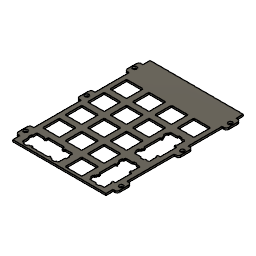
Plate (Autodesk Fusion 360 design; units mm, degrees)
part number: 2026-08-19-10-44-33-634
Autodesk Fusion 360 part; units mm, degrees
sketch "plate-2026-08-19T09_43_30.871Z" plane through (0, 0, 0) normal (0, 0, 1) x (1, 0, 0)
  line L0 (3.025, -2.525) -> (16.025, -2.525)
  line L1 (3.025, -16.525) -> (16.025, -16.525)
  line L2 (2.525, -3.025) -> (2.525, -16.025)
  line L3 (16.525, -3.025) -> (16.525, -16.025)
  arc A0 (3.025, -2.525) -> (2.525, -3.025) centre (3.025, -3.025) ccw
  arc A1 (16.525, -3.025) -> (16.025, -2.525) centre (16.025, -3.025) ccw
  arc A2 (2.525, -16.025) -> (3.025, -16.525) centre (3.025, -16.025) ccw
  arc A3 (16.025, -16.525) -> (16.525, -16.025) centre (16.025, -16.025) ccw
  line L4 (22.075, -2.525) -> (35.075, -2.525)
  line L5 (22.075, -16.525) -> (35.075, -16.525)
  line L6 (21.575, -3.025) -> (21.575, -16.025)
  line L7 (35.575, -3.025) -> (35.575, -16.025)
  arc A4 (22.075, -2.525) -> (21.575, -3.025) centre (22.075, -3.025) ccw
  arc A5 (35.575, -3.025) -> (35.075, -2.525) centre (35.075, -3.025) ccw
  arc A6 (21.575, -16.025) -> (22.075, -16.525) centre (22.075, -16.025) ccw
  arc A7 (35.075, -16.525) -> (35.575, -16.025) centre (35.075, -16.025) ccw
  line L8 (41.125, -2.525) -> (54.125, -2.525)
  line L9 (41.125, -16.525) -> (54.125, -16.525)
  line L10 (40.625, -3.025) -> (40.625, -16.025)
  line L11 (54.625, -3.025) -> (54.625, -16.025)
  arc A8 (41.125, -2.525) -> (40.625, -3.025) centre (41.125, -3.025) ccw
  arc A9 (54.625, -3.025) -> (54.125, -2.525) centre (54.125, -3.025) ccw
  arc A10 (40.625, -16.025) -> (41.125, -16.525) centre (41.125, -16.025) ccw
  arc A11 (54.125, -16.525) -> (54.625, -16.025) centre (54.125, -16.025) ccw
  line L12 (60.175, -2.525) -> (73.175, -2.525)
  line L13 (60.175, -16.525) -> (73.175, -16.525)
  line L14 (59.675, -3.025) -> (59.675, -16.025)
  line L15 (73.675, -3.025) -> (73.675, -16.025)
  arc A12 (60.175, -2.525) -> (59.675, -3.025) centre (60.175, -3.025) ccw
  arc A13 (73.675, -3.025) -> (73.175, -2.525) centre (73.175, -3.025) ccw
  arc A14 (59.675, -16.025) -> (60.175, -16.525) centre (60.175, -16.025) ccw
  arc A15 (73.175, -16.525) -> (73.675, -16.025) centre (73.175, -16.025) ccw
  line L16 (3.025, -21.575) -> (16.025, -21.575)
  line L17 (3.025, -35.575) -> (16.025, -35.575)
  line L18 (2.525, -22.075) -> (2.525, -35.075)
  line L19 (16.525, -22.075) -> (16.525, -35.075)
  arc A16 (3.025, -21.575) -> (2.525, -22.075) centre (3.025, -22.075) ccw
  arc A17 (16.525, -22.075) -> (16.025, -21.575) centre (16.025, -22.075) ccw
  arc A18 (2.525, -35.075) -> (3.025, -35.575) centre (3.025, -35.075) ccw
  arc A19 (16.025, -35.575) -> (16.525, -35.075) centre (16.025, -35.075) ccw
  line L20 (22.075, -21.575) -> (35.075, -21.575)
  line L21 (22.075, -35.575) -> (35.075, -35.575)
  line L22 (21.575, -22.075) -> (21.575, -35.075)
  line L23 (35.575, -22.075) -> (35.575, -35.075)
  arc A20 (22.075, -21.575) -> (21.575, -22.075) centre (22.075, -22.075) ccw
  arc A21 (35.575, -22.075) -> (35.075, -21.575) centre (35.075, -22.075) ccw
  arc A22 (21.575, -35.075) -> (22.075, -35.575) centre (22.075, -35.075) ccw
  arc A23 (35.075, -35.575) -> (35.575, -35.075) centre (35.075, -35.075) ccw
  line L24 (41.125, -21.575) -> (54.125, -21.575)
  line L25 (41.125, -35.575) -> (54.125, -35.575)
  line L26 (40.625, -22.075) -> (40.625, -35.075)
  line L27 (54.625, -22.075) -> (54.625, -35.075)
  arc A24 (41.125, -21.575) -> (40.625, -22.075) centre (41.125, -22.075) ccw
  arc A25 (54.625, -22.075) -> (54.125, -21.575) centre (54.125, -22.075) ccw
  arc A26 (40.625, -35.075) -> (41.125, -35.575) centre (41.125, -35.075) ccw
  arc A27 (54.125, -35.575) -> (54.625, -35.075) centre (54.125, -35.075) ccw
  line L28 (73.675, -31.6) -> (73.675, -44.6)
  line L29 (59.675, -31.6) -> (59.675, -44.6)
  line L30 (73.175, -31.1) -> (60.175, -31.1)
  line L31 (73.175, -45.1) -> (60.175, -45.1)
  arc A28 (73.675, -31.6) -> (73.175, -31.1) centre (73.175, -31.6) ccw
  arc A29 (73.175, -45.1) -> (73.675, -44.6) centre (73.175, -44.6) ccw
  arc A30 (60.175, -31.1) -> (59.675, -31.6) centre (60.175, -31.6) ccw
  arc A31 (59.675, -44.6) -> (60.175, -45.1) centre (60.175, -44.6) ccw
  line L32 (72.3646, -23.3346) -> (72.3646, -28.9894)
  line L33 (71.8646, -29.4894) -> (71.5518, -29.4894)
  line L34 (71.5518, -29.4894) -> (71.5518, -38.1)
  line L35 (60.8584, -38.1) -> (60.8584, -29.9894)
  line L36 (60.3584, -29.4894) -> (60.071, -29.4894)
  line L37 (60.071, -29.4894) -> (60.071, -28.186)
  line L38 (59.571, -27.686) -> (59.4026, -27.686)
  line L39 (58.9026, -27.186) -> (58.9026, -25.138)
  line L40 (59.4026, -24.638) -> (59.571, -24.638)
  line L41 (60.071, -24.138) -> (60.071, -23.3346)
  line L42 (60.571, -22.8346) -> (65.667, -22.8346)
  line L43 (66.167, -22.3346) -> (66.167, -21.971)
  line L44 (66.167, -21.971) -> (68.461, -21.971)
  line L45 (68.961, -22.471) -> (68.961, -22.8346)
  line L46 (68.961, -22.8346) -> (71.8646, -22.8346)
  arc A32 (71.8646, -29.4894) -> (72.3646, -28.9894) centre (71.8646, -28.9894) ccw
  arc A33 (60.8584, -29.9894) -> (60.3584, -29.4894) centre (60.3584, -29.9894) ccw
  arc A34 (60.071, -28.186) -> (59.571, -27.686) centre (59.571, -28.186) ccw
  arc A35 (58.9026, -27.186) -> (59.4026, -27.686) centre (59.4026, -27.186) ccw
  arc A36 (59.4026, -24.638) -> (58.9026, -25.138) centre (59.4026, -25.138) ccw
  arc A37 (59.571, -24.638) -> (60.071, -24.138) centre (59.571, -24.138) ccw
  arc A38 (60.571, -22.8346) -> (60.071, -23.3346) centre (60.571, -23.3346) ccw
  arc A39 (65.667, -22.8346) -> (66.167, -22.3346) centre (65.667, -22.3346) ccw
  arc A40 (68.961, -22.471) -> (68.461, -21.971) centre (68.461, -22.471) ccw
  arc A41 (72.3646, -23.3346) -> (71.8646, -22.8346) centre (71.8646, -23.3346) ccw
  line L47 (72.3646, -52.8654) -> (72.3646, -47.2106)
  line L48 (71.8646, -46.7106) -> (71.5518, -46.7106)
  line L49 (71.5518, -46.7106) -> (71.5518, -38.1)
  line L50 (60.8584, -38.1) -> (60.8584, -46.2106)
  line L51 (60.3584, -46.7106) -> (60.071, -46.7106)
  line L52 (60.071, -46.7106) -> (60.071, -48.014)
  line L53 (59.571, -48.514) -> (59.4026, -48.514)
  line L54 (58.9026, -49.014) -> (58.9026, -51.062)
  line L55 (59.4026, -51.562) -> (59.571, -51.562)
  line L56 (60.071, -52.062) -> (60.071, -52.8654)
  line L57 (60.571, -53.3654) -> (65.667, -53.3654)
  line L58 (66.167, -53.8654) -> (66.167, -54.229)
  line L59 (66.167, -54.229) -> (68.461, -54.229)
  line L60 (68.961, -53.729) -> (68.961, -53.3654)
  line L61 (68.961, -53.3654) -> (71.8646, -53.3654)
  arc A42 (72.3646, -47.2106) -> (71.8646, -46.7106) centre (71.8646, -47.2106) ccw
  arc A43 (60.3584, -46.7106) -> (60.8584, -46.2106) centre (60.3584, -46.2106) ccw
  arc A44 (59.571, -48.514) -> (60.071, -48.014) centre (59.571, -48.014) ccw
  arc A45 (59.4026, -48.514) -> (58.9026, -49.014) centre (59.4026, -49.014) ccw
  arc A46 (58.9026, -51.062) -> (59.4026, -51.562) centre (59.4026, -51.062) ccw
  arc A47 (60.071, -52.062) -> (59.571, -51.562) centre (59.571, -52.062) ccw
  arc A48 (60.071, -52.8654) -> (60.571, -53.3654) centre (60.571, -52.8654) ccw
  arc A49 (66.167, -53.8654) -> (65.667, -53.3654) centre (65.667, -53.8654) ccw
  arc A50 (68.461, -54.229) -> (68.961, -53.729) centre (68.461, -53.729) ccw
  arc A51 (71.8646, -53.3654) -> (72.3646, -52.8654) centre (71.8646, -52.8654) ccw
  line L62 (3.025, -40.625) -> (16.025, -40.625)
  line L63 (3.025, -54.625) -> (16.025, -54.625)
  line L64 (2.525, -41.125) -> (2.525, -54.125)
  line L65 (16.525, -41.125) -> (16.525, -54.125)
  arc A52 (3.025, -40.625) -> (2.525, -41.125) centre (3.025, -41.125) ccw
  arc A53 (16.525, -41.125) -> (16.025, -40.625) centre (16.025, -41.125) ccw
  arc A54 (2.525, -54.125) -> (3.025, -54.625) centre (3.025, -54.125) ccw
  arc A55 (16.025, -54.625) -> (16.525, -54.125) centre (16.025, -54.125) ccw
  line L66 (22.075, -40.625) -> (35.075, -40.625)
  line L67 (22.075, -54.625) -> (35.075, -54.625)
  line L68 (21.575, -41.125) -> (21.575, -54.125)
  line L69 (35.575, -41.125) -> (35.575, -54.125)
  arc A56 (22.075, -40.625) -> (21.575, -41.125) centre (22.075, -41.125) ccw
  arc A57 (35.575, -41.125) -> (35.075, -40.625) centre (35.075, -41.125) ccw
  arc A58 (21.575, -54.125) -> (22.075, -54.625) centre (22.075, -54.125) ccw
  arc A59 (35.075, -54.625) -> (35.575, -54.125) centre (35.075, -54.125) ccw
  line L70 (41.125, -40.625) -> (54.125, -40.625)
  line L71 (41.125, -54.625) -> (54.125, -54.625)
  line L72 (40.625, -41.125) -> (40.625, -54.125)
  line L73 (54.625, -41.125) -> (54.625, -54.125)
  arc A60 (41.125, -40.625) -> (40.625, -41.125) centre (41.125, -41.125) ccw
  arc A61 (54.625, -41.125) -> (54.125, -40.625) centre (54.125, -41.125) ccw
  arc A62 (40.625, -54.125) -> (41.125, -54.625) centre (41.125, -54.125) ccw
  arc A63 (54.125, -54.625) -> (54.625, -54.125) centre (54.125, -54.125) ccw
  line L74 (3.025, -59.675) -> (16.025, -59.675)
  line L75 (3.025, -73.675) -> (16.025, -73.675)
  line L76 (2.525, -60.175) -> (2.525, -73.175)
  line L77 (16.525, -60.175) -> (16.525, -73.175)
  arc A64 (3.025, -59.675) -> (2.525, -60.175) centre (3.025, -60.175) ccw
  arc A65 (16.525, -60.175) -> (16.025, -59.675) centre (16.025, -60.175) ccw
  arc A66 (2.525, -73.175) -> (3.025, -73.675) centre (3.025, -73.175) ccw
  arc A67 (16.025, -73.675) -> (16.525, -73.175) centre (16.025, -73.175) ccw
  line L78 (22.075, -59.675) -> (35.075, -59.675)
  line L79 (22.075, -73.675) -> (35.075, -73.675)
  line L80 (21.575, -60.175) -> (21.575, -73.175)
  line L81 (35.575, -60.175) -> (35.575, -73.175)
  arc A68 (22.075, -59.675) -> (21.575, -60.175) centre (22.075, -60.175) ccw
  arc A69 (35.575, -60.175) -> (35.075, -59.675) centre (35.075, -60.175) ccw
  arc A70 (21.575, -73.175) -> (22.075, -73.675) centre (22.075, -73.175) ccw
  arc A71 (35.075, -73.675) -> (35.575, -73.175) centre (35.075, -73.175) ccw
  line L82 (41.125, -59.675) -> (54.125, -59.675)
  line L83 (41.125, -73.675) -> (54.125, -73.675)
  line L84 (40.625, -60.175) -> (40.625, -73.175)
  line L85 (54.625, -60.175) -> (54.625, -73.175)
  arc A72 (41.125, -59.675) -> (40.625, -60.175) centre (41.125, -60.175) ccw
  arc A73 (54.625, -60.175) -> (54.125, -59.675) centre (54.125, -60.175) ccw
  arc A74 (40.625, -73.175) -> (41.125, -73.675) centre (41.125, -73.175) ccw
  arc A75 (54.125, -73.675) -> (54.625, -73.175) centre (54.125, -73.175) ccw
  line L86 (73.675, -69.7) -> (73.675, -82.7)
  line L87 (59.675, -69.7) -> (59.675, -82.7)
  line L88 (73.175, -69.2) -> (60.175, -69.2)
  line L89 (73.175, -83.2) -> (60.175, -83.2)
  arc A76 (73.675, -69.7) -> (73.175, -69.2) centre (73.175, -69.7) ccw
  arc A77 (73.175, -83.2) -> (73.675, -82.7) centre (73.175, -82.7) ccw
  arc A78 (60.175, -69.2) -> (59.675, -69.7) centre (60.175, -69.7) ccw
  arc A79 (59.675, -82.7) -> (60.175, -83.2) centre (60.175, -82.7) ccw
  line L90 (72.3646, -61.4346) -> (72.3646, -67.0894)
  line L91 (71.8646, -67.5894) -> (71.5518, -67.5894)
  line L92 (71.5518, -67.5894) -> (71.5518, -76.2)
  line L93 (60.8584, -76.2) -> (60.8584, -68.0894)
  line L94 (60.3584, -67.5894) -> (60.071, -67.5894)
  line L95 (60.071, -67.5894) -> (60.071, -66.286)
  line L96 (59.571, -65.786) -> (59.4026, -65.786)
  line L97 (58.9026, -65.286) -> (58.9026, -63.238)
  line L98 (59.4026, -62.738) -> (59.571, -62.738)
  line L99 (60.071, -62.238) -> (60.071, -61.4346)
  line L100 (60.571, -60.9346) -> (65.667, -60.9346)
  line L101 (66.167, -60.4346) -> (66.167, -60.071)
  line L102 (66.167, -60.071) -> (68.461, -60.071)
  line L103 (68.961, -60.571) -> (68.961, -60.9346)
  line L104 (68.961, -60.9346) -> (71.8646, -60.9346)
  arc A80 (71.8646, -67.5894) -> (72.3646, -67.0894) centre (71.8646, -67.0894) ccw
  arc A81 (60.8584, -68.0894) -> (60.3584, -67.5894) centre (60.3584, -68.0894) ccw
  arc A82 (60.071, -66.286) -> (59.571, -65.786) centre (59.571, -66.286) ccw
  arc A83 (58.9026, -65.286) -> (59.4026, -65.786) centre (59.4026, -65.286) ccw
  arc A84 (59.4026, -62.738) -> (58.9026, -63.238) centre (59.4026, -63.238) ccw
  arc A85 (59.571, -62.738) -> (60.071, -62.238) centre (59.571, -62.238) ccw
  arc A86 (60.571, -60.9346) -> (60.071, -61.4346) centre (60.571, -61.4346) ccw
  arc A87 (65.667, -60.9346) -> (66.167, -60.4346) centre (65.667, -60.4346) ccw
  arc A88 (68.961, -60.571) -> (68.461, -60.071) centre (68.461, -60.571) ccw
  arc A89 (72.3646, -61.4346) -> (71.8646, -60.9346) centre (71.8646, -61.4346) ccw
  line L105 (72.3646, -90.9654) -> (72.3646, -85.3106)
  line L106 (71.8646, -84.8106) -> (71.5518, -84.8106)
  line L107 (71.5518, -84.8106) -> (71.5518, -76.2)
  line L108 (60.8584, -76.2) -> (60.8584, -84.3106)
  line L109 (60.3584, -84.8106) -> (60.071, -84.8106)
  line L110 (60.071, -84.8106) -> (60.071, -86.114)
  line L111 (59.571, -86.614) -> (59.4026, -86.614)
  line L112 (58.9026, -87.114) -> (58.9026, -89.162)
  line L113 (59.4026, -89.662) -> (59.571, -89.662)
  line L114 (60.071, -90.162) -> (60.071, -90.9654)
  line L115 (60.571, -91.4654) -> (65.667, -91.4654)
  line L116 (66.167, -91.9654) -> (66.167, -92.329)
  line L117 (66.167, -92.329) -> (68.461, -92.329)
  line L118 (68.961, -91.829) -> (68.961, -91.4654)
  line L119 (68.961, -91.4654) -> (71.8646, -91.4654)
  arc A90 (72.3646, -85.3106) -> (71.8646, -84.8106) centre (71.8646, -85.3106) ccw
  arc A91 (60.3584, -84.8106) -> (60.8584, -84.3106) centre (60.3584, -84.3106) ccw
  arc A92 (59.571, -86.614) -> (60.071, -86.114) centre (59.571, -86.114) ccw
  arc A93 (59.4026, -86.614) -> (58.9026, -87.114) centre (59.4026, -87.114) ccw
  arc A94 (58.9026, -89.162) -> (59.4026, -89.662) centre (59.4026, -89.162) ccw
  arc A95 (60.071, -90.162) -> (59.571, -89.662) centre (59.571, -90.162) ccw
  arc A96 (60.071, -90.9654) -> (60.571, -91.4654) centre (60.571, -90.9654) ccw
  arc A97 (66.167, -91.9654) -> (65.667, -91.4654) centre (65.667, -91.9654) ccw
  arc A98 (68.461, -92.329) -> (68.961, -91.829) centre (68.461, -91.829) ccw
  arc A99 (71.8646, -91.4654) -> (72.3646, -90.9654) centre (71.8646, -90.9654) ccw
  line L120 (12.55, -78.725) -> (25.55, -78.725)
  line L121 (12.55, -92.725) -> (25.55, -92.725)
  line L122 (12.05, -79.225) -> (12.05, -92.225)
  line L123 (26.05, -79.225) -> (26.05, -92.225)
  arc A100 (12.55, -78.725) -> (12.05, -79.225) centre (12.55, -79.225) ccw
  arc A101 (26.05, -79.225) -> (25.55, -78.725) centre (25.55, -79.225) ccw
  arc A102 (12.05, -92.225) -> (12.55, -92.725) centre (12.55, -92.225) ccw
  arc A103 (25.55, -92.725) -> (26.05, -92.225) centre (25.55, -92.225) ccw
  line L124 (4.2846, -80.0354) -> (9.9394, -80.0354)
  line L125 (10.4394, -80.5354) -> (10.4394, -80.8482)
  line L126 (10.4394, -80.8482) -> (19.05, -80.8482)
  line L127 (19.05, -91.5416) -> (10.9394, -91.5416)
  line L128 (10.4394, -92.0416) -> (10.4394, -92.329)
  line L129 (10.4394, -92.329) -> (9.136, -92.329)
  line L130 (8.636, -92.829) -> (8.636, -92.9974)
  line L131 (8.136, -93.4974) -> (6.088, -93.4974)
  line L132 (5.588, -92.9974) -> (5.588, -92.829)
  line L133 (5.088, -92.329) -> (4.2846, -92.329)
  line L134 (3.7846, -91.829) -> (3.7846, -86.733)
  line L135 (3.2846, -86.233) -> (2.921, -86.233)
  line L136 (2.921, -86.233) -> (2.921, -83.939)
  line L137 (3.421, -83.439) -> (3.7846, -83.439)
  line L138 (3.7846, -83.439) -> (3.7846, -80.5354)
  arc A104 (10.4394, -80.5354) -> (9.9394, -80.0354) centre (9.9394, -80.5354) ccw
  arc A105 (10.9394, -91.5416) -> (10.4394, -92.0416) centre (10.9394, -92.0416) ccw
  arc A106 (9.136, -92.329) -> (8.636, -92.829) centre (9.136, -92.829) ccw
  arc A107 (8.136, -93.4974) -> (8.636, -92.9974) centre (8.136, -92.9974) ccw
  arc A108 (5.588, -92.9974) -> (6.088, -93.4974) centre (6.088, -92.9974) ccw
  arc A109 (5.588, -92.829) -> (5.088, -92.329) centre (5.088, -92.829) ccw
  arc A110 (3.7846, -91.829) -> (4.2846, -92.329) centre (4.2846, -91.829) ccw
  arc A111 (3.7846, -86.733) -> (3.2846, -86.233) centre (3.2846, -86.733) ccw
  arc A112 (3.421, -83.439) -> (2.921, -83.939) centre (3.421, -83.939) ccw
  arc A113 (4.2846, -80.0354) -> (3.7846, -80.5354) centre (4.2846, -80.5354) ccw
  line L139 (33.8154, -80.0354) -> (28.1606, -80.0354)
  line L140 (27.6606, -80.5354) -> (27.6606, -80.8482)
  line L141 (27.6606, -80.8482) -> (19.05, -80.8482)
  line L142 (19.05, -91.5416) -> (27.1606, -91.5416)
  line L143 (27.6606, -92.0416) -> (27.6606, -92.329)
  line L144 (27.6606, -92.329) -> (28.964, -92.329)
  line L145 (29.464, -92.829) -> (29.464, -92.9974)
  line L146 (29.964, -93.4974) -> (32.012, -93.4974)
  line L147 (32.512, -92.9974) -> (32.512, -92.829)
  line L148 (33.012, -92.329) -> (33.8154, -92.329)
  line L149 (34.3154, -91.829) -> (34.3154, -86.733)
  line L150 (34.8154, -86.233) -> (35.179, -86.233)
  line L151 (35.179, -86.233) -> (35.179, -83.939)
  line L152 (34.679, -83.439) -> (34.3154, -83.439)
  line L153 (34.3154, -83.439) -> (34.3154, -80.5354)
  arc A114 (28.1606, -80.0354) -> (27.6606, -80.5354) centre (28.1606, -80.5354) ccw
  arc A115 (27.6606, -92.0416) -> (27.1606, -91.5416) centre (27.1606, -92.0416) ccw
  arc A116 (29.464, -92.829) -> (28.964, -92.329) centre (28.964, -92.829) ccw
  arc A117 (29.464, -92.9974) -> (29.964, -93.4974) centre (29.964, -92.9974) ccw
  arc A118 (32.012, -93.4974) -> (32.512, -92.9974) centre (32.012, -92.9974) ccw
  arc A119 (33.012, -92.329) -> (32.512, -92.829) centre (33.012, -92.829) ccw
  arc A120 (33.8154, -92.329) -> (34.3154, -91.829) centre (33.8154, -91.829) ccw
  arc A121 (34.8154, -86.233) -> (34.3154, -86.733) centre (34.8154, -86.733) ccw
  arc A122 (35.179, -83.939) -> (34.679, -83.439) centre (34.679, -83.939) ccw
  arc A123 (34.3154, -80.5354) -> (33.8154, -80.0354) centre (33.8154, -80.5354) ccw
  line L154 (41.125, -78.725) -> (54.125, -78.725)
  line L155 (41.125, -92.725) -> (54.125, -92.725)
  line L156 (40.625, -79.225) -> (40.625, -92.225)
  line L157 (54.625, -79.225) -> (54.625, -92.225)
  arc A124 (41.125, -78.725) -> (40.625, -79.225) centre (41.125, -79.225) ccw
  arc A125 (54.625, -79.225) -> (54.125, -78.725) centre (54.125, -79.225) ccw
  arc A126 (40.625, -92.225) -> (41.125, -92.725) centre (41.125, -92.225) ccw
  arc A127 (54.125, -92.725) -> (54.625, -92.225) centre (54.125, -92.225) ccw
  line L158 (0, -95.25) -> (76.2, -95.25)
  line L159 (0, 0) -> (76.2, 0)
  line L160 (0, -95.25) -> (0, 0)
  line L161 (76.2, -95.25) -> (76.2, 0)
sketch "Sketch2" plane through (0, 0, 0) normal (0, 0, 1) x (1, 0, 0)
  line L0 (0, -95.25) -> (76.2, -95.25)
  line L1 (76.2, -95.25) -> (76.2, 0)
  line L2 (0, -95.25) -> (0, 0)
  line L3 (76.2, 21.431) -> (0, 21.431)
  line L4 (0, 0) -> (76.2, 0)
  line L5 (0, 0) -> (0, 21.431)
  line L6 (0, -95.25) -> (76.2, -95.25)
  line L7 (76.2, -95.25) -> (76.2, 0)
  line L8 (76.2, 21.431) -> (76.2, -95.25)
  line L9 (0, 21.431) -> (0, -95.25)
  dimension "d1" = 21.431
  constraint perpendicular L2 L3
  constraint coincident L2.end L4.start
  constraint perpendicular L3 L5
  constraint coincident L0.start L2.start
  constraint coincident L0.end L1.start
  constraint coincident L1.end L4.end
  constraint perpendicular L6 L8
  measures "d1" distance of L3 L4
sketch "Sketch3" plane through (0, 0, 0) normal (0, 0, 1) x (1, 0, 0)
  line L0 (0, 21.431) -> (0, -95.25)
  line L1 (76.2, 21.431) -> (76.2, -95.25)
  line L2 (76.2, 21.431) -> (0, 21.431)
  line L3 (0, -95.25) -> (76.2, -95.25)
  line L4 (81.2, -95.25) -> (-5, -95.25)
  line L5 (-5, 21.431) -> (81.2, 21.431)
  line L6 (76.2, 21.431) -> (82.6, 21.431)
  line L7 (82.6, 21.431) -> (82.6, -95.25)
  line L8 (82.6, -95.25) -> (76.2, -95.25)
  line L9 (76.2, -95.25) -> (76.2, 0)
  line L10 (0, 21.431) -> (-6.4, 21.431)
  line L11 (-6.4, 21.431) -> (-6.4, -95.25)
  line L12 (-6.4, -95.25) -> (0, -95.25)
  line L13 (-3, 15.431) -> (0, 15.431)
  line L14 (0, 3.431) -> (-3, 3.431)
  line L15 (-5, 5.431) -> (-5, 13.431)
  circle A0 centre (-2.5, 9.431) radius 1.7
  line L16 (76.2, 15.431) -> (79.2, 15.431)
  line L17 (81.2, 13.431) -> (81.2, 5.431)
  line L18 (79.2, 3.431) -> (76.2, 3.431)
  circle A1 centre (78.7, 9.431) radius 1.7
  line L19 (0, -89.25) -> (-3, -89.25)
  line L20 (-5, -87.25) -> (-5, -79.25)
  line L21 (-3, -77.25) -> (0, -77.25)
  line L22 (76.2, -89.25) -> (79.2, -89.25)
  line L23 (81.2, -87.25) -> (81.2, -79.25)
  line L24 (79.2, -77.25) -> (76.2, -77.25)
  line L25 (76.2, -77.25) -> (76.2, -89.25)
  circle A2 centre (78.7, -83.25) radius 1.7
  circle A3 centre (-2.5, -83.25) radius 1.7
  line L26 (76.2, -25.25) -> (79.2, -25.25)
  line L27 (81.2, -27.25) -> (81.2, -35.25)
  line L28 (79.2, -37.25) -> (76.2, -37.25)
  circle A4 centre (78.7, -31.25) radius 1.7
  line L29 (0, -37.25) -> (-3, -37.25)
  line L30 (-5, -35.25) -> (-5, -27.25)
  line L31 (-3, -25.25) -> (0, -25.25)
  circle A5 centre (-2.5, -31.25) radius 1.7
  line L32 (81.2, 13.431) -> (81.2, 5.431)
  line L33 (81.2, -27.25) -> (81.2, -35.25)
  line L34 (81.2, -79.25) -> (81.2, -87.25)
  line L35 (-5, -87.25) -> (-5, -79.25)
  line L36 (-5, -35.25) -> (-5, -27.25)
  arc A6 (-3, 15.431) -> (-5, 13.431) centre (-3, 13.431) ccw
  arc A7 (-5, 5.431) -> (-3, 3.431) centre (-3, 5.431) ccw
  arc A8 (-3, -25.25) -> (-5, -27.25) centre (-3, -27.25) ccw
  arc A9 (-5, -35.25) -> (-3, -37.25) centre (-3, -35.25) ccw
  arc A10 (-3, -77.25) -> (-5, -79.25) centre (-3, -79.25) ccw
  arc A11 (-5, -87.25) -> (-3, -89.25) centre (-3, -87.25) ccw
  arc A12 (79.2, -89.25) -> (81.2, -87.25) centre (79.2, -87.25) ccw
  arc A13 (81.2, -79.25) -> (79.2, -77.25) centre (79.2, -79.25) ccw
  arc A14 (79.2, -37.25) -> (81.2, -35.25) centre (79.2, -35.25) ccw
  arc A15 (81.2, -27.25) -> (79.2, -25.25) centre (79.2, -27.25) ccw
  arc A16 (79.2, 3.431) -> (81.2, 5.431) centre (79.2, 5.431) ccw
  arc A17 (81.2, 13.431) -> (79.2, 15.431) centre (79.2, 13.431) ccw
  line L37 (76.2, -95.25) -> (76.2, -37.25)
  line L38 (76.2, -25.25) -> (76.2, 3.431)
  line L39 (76.2, 15.431) -> (76.2, 21.431)
  line L40 (0, 15.431) -> (0, 21.431)
  line L41 (0, -25.25) -> (0, 3.431)
  line L42 (0, -95.25) -> (0, -89.25)
  line L43 (0, -77.25) -> (0, -37.25)
  dimension "d2" = 5
  dimension "d3" = 5
  dimension "d4" = 6.4
  dimension "d5" = 6.4
  dimension "d6" = 12
  dimension "d7" = 6
  dimension "d8" = 3.4
  dimension "d9" = 2.5
  dimension "d10" = 6
  dimension "d11" = 12
  dimension "d12" = 3.4
  dimension "d13" = 2.5
  dimension "d14" = 6
  dimension "d15" = 6
  dimension "d16" = 12
  dimension "d17" = 12
  dimension "d18" = 6
  dimension "d19" = 6
  dimension "d20" = 3.4
  dimension "d21" = 2.5
  dimension "d22" = 6
  dimension "d23" = 3.4
  dimension "d24" = 6
  dimension "d25" = 2.5
  dimension "d26" = 12
  dimension "d27" = 3.4
  dimension "d28" = 12
  dimension "d29" = 3.4
  dimension "d30" = 2.5
  dimension "d31" = 6
  dimension "d32" = 2.5
  dimension "d33" = 6
  dimension "d34" = 40
  dimension "d35" = 40
  dimension "d36" = 2
  constraint horizontal L4
  constraint vertical L35
  constraint horizontal L5
  constraint vertical L32
  constraint horizontal L6
  constraint vertical L7
  constraint horizontal L8
  constraint vertical L37
  constraint coincident L1.start L2.start
  constraint horizontal L10
  constraint vertical L11
  constraint horizontal L12
  constraint vertical L42
  constraint coincident L0.start L2.end
  constraint horizontal L13
  constraint horizontal L14
  constraint vertical L15
  constraint horizontal L16
  constraint vertical L17
  constraint horizontal L18
  constraint coincident L1 L16.start
  constraint horizontal L19
  constraint vertical L20
  constraint horizontal L21
  constraint coincident L0 L19.start
  constraint horizontal L22
  constraint vertical L23
  constraint horizontal L24
  constraint vertical L25
  constraint coincident L1 L22.start
  constraint horizontal L26
  constraint vertical L27
  constraint horizontal L28
  constraint horizontal L29
  constraint vertical L30
  constraint horizontal L31
  constraint collinear L32 L33
  constraint collinear L33 L34
  constraint collinear L35 L36
  constraint tangent L15 A6
  constraint tangent L13 A6
  constraint tangent L15 A7
  constraint tangent L14 A7
  constraint equal A6 A7
  constraint tangent L31 A8
  constraint tangent L36 A8
  constraint equal A6 A8
  constraint tangent L29 A9
  constraint tangent L30 A9
  constraint equal A6 A9
  constraint tangent L21 A10
  constraint tangent L20 A10
  constraint equal A6 A10
  constraint tangent L19 A11
  constraint tangent L35 A11
  constraint equal A6 A11
  constraint tangent L22 A12
  constraint tangent L23 A12
  constraint equal A6 A12
  constraint tangent L24 A13
  constraint tangent L34 A13
  constraint equal A6 A13
  constraint tangent L28 A14
  constraint tangent L27 A14
  constraint equal A6 A14
  constraint tangent L26 A15
  constraint tangent L33 A15
  constraint equal A6 A15
  constraint tangent L18 A16
  constraint tangent L32 A16
  constraint equal A6 A16
  constraint tangent L16 A17
  constraint tangent L17 A17
  constraint equal A6 A17
  constraint collinear L37 L38
  constraint collinear L38 L39
  constraint collinear L40 L41
  constraint collinear L41 L43
  constraint collinear L42 L43
  measures "d2" distance of L0 L35
  measures "d3" distance of L1 L32
  measures "d4" distance of L7 L9
  measures "d5" distance of L0 L11
  measures "d6" distance of L13 L14
  measures "d7" distance of L5 L13
  measures "d8" diameter of A0
  measures "d9" distance of L0 A0.centre
  measures "d10" distance of L5 L16
  measures "d11" distance of L16 L18
  measures "d12" diameter of A1
  measures "d13" distance of L1 A1.centre
  measures "d14" distance of L16 A1.centre
  measures "d15" distance of L13 A0.centre
  measures "d16" distance of L22 L24
  measures "d17" distance of L19 L21
  measures "d18" distance of L4 L19
  measures "d19" distance of L4 L22
  measures "d20" diameter of A2
  measures "d21" distance of L1 A2.centre
  measures "d22" distance of L22 A2.centre
  measures "d23" diameter of A3
  measures "d24" distance of L19 A3.centre
  measures "d25" distance of L0 A3.centre
  measures "d26" distance of L26 L28
  measures "d27" diameter of A4
  measures "d28" distance of L29 L31
  measures "d29" diameter of A5
  measures "d30" distance of L9 A4.centre
  measures "d31" distance of L28 A4.centre
  measures "d32" distance of L0 A5.centre
  measures "d33" distance of L31 A5.centre
  measures "d34" distance of L21 L29
  measures "d35" distance of L24 L28
  measures "d36" radius of A6
sketch "Sketch4" plane through (0, 0, 0) normal (0, 0, 1) x (1, 0, 0)
  line L0 (3.025, -2.525) -> (16.025, -2.525)
  line L1 (2.525, -3.025) -> (2.525, -16.025)
  line L2 (16.525, -3.025) -> (16.525, -16.025)
  arc A0 (16.525, -3.025) -> (16.025, -2.525) centre (16.025, -3.025) ccw
  arc A1 (3.025, -2.525) -> (2.525, -3.025) centre (3.025, -3.025) ccw
  arc A2 (2.525, -16.025) -> (3.025, -16.525) centre (3.025, -16.025) ccw
  line L3 (3.025, -16.525) -> (16.025, -16.525)
  arc A3 (16.025, -16.525) -> (16.525, -16.025) centre (16.025, -16.025) ccw
  line L4 (22.075, -16.525) -> (35.075, -16.525)
  arc A4 (21.575, -16.025) -> (22.075, -16.525) centre (22.075, -16.025) ccw
  line L5 (21.575, -3.025) -> (21.575, -16.025)
  arc A5 (35.075, -16.525) -> (35.575, -16.025) centre (35.075, -16.025) ccw
  line L6 (35.575, -3.025) -> (35.575, -16.025)
  line L7 (22.075, -2.525) -> (35.075, -2.525)
  arc A6 (35.575, -3.025) -> (35.075, -2.525) centre (35.075, -3.025) ccw
  arc A7 (22.075, -2.525) -> (21.575, -3.025) centre (22.075, -3.025) ccw
  arc A8 (41.125, -2.525) -> (40.625, -3.025) centre (41.125, -3.025) ccw
  line L8 (40.625, -3.025) -> (40.625, -16.025)
  line L9 (41.125, -2.525) -> (54.125, -2.525)
  arc A9 (40.625, -16.025) -> (41.125, -16.525) centre (41.125, -16.025) ccw
  line L10 (41.125, -16.525) -> (54.125, -16.525)
  line L11 (54.625, -3.025) -> (54.625, -16.025)
  arc A10 (54.125, -16.525) -> (54.625, -16.025) centre (54.125, -16.025) ccw
  arc A11 (54.625, -3.025) -> (54.125, -2.525) centre (54.125, -3.025) ccw
  arc A12 (60.175, -2.525) -> (59.675, -3.025) centre (60.175, -3.025) ccw
  line L12 (59.675, -3.025) -> (59.675, -16.025)
  line L13 (60.175, -2.525) -> (73.175, -2.525)
  arc A13 (59.675, -16.025) -> (60.175, -16.525) centre (60.175, -16.025) ccw
  line L14 (60.175, -16.525) -> (73.175, -16.525)
  arc A14 (73.175, -16.525) -> (73.675, -16.025) centre (73.175, -16.025) ccw
  line L15 (73.675, -3.025) -> (73.675, -16.025)
  arc A15 (73.675, -3.025) -> (73.175, -2.525) centre (73.175, -3.025) ccw
  line L16 (66.167, -21.971) -> (68.461, -21.971)
  arc A16 (65.667, -22.8346) -> (66.167, -22.3346) centre (65.667, -22.3346) ccw
  line L17 (66.167, -22.3346) -> (66.167, -21.971)
  arc A17 (68.961, -22.471) -> (68.461, -21.971) centre (68.461, -22.471) ccw
  line L18 (68.961, -22.471) -> (68.961, -22.8346)
  line L19 (68.961, -22.8346) -> (71.8646, -22.8346)
  arc A18 (72.3646, -23.3346) -> (71.8646, -22.8346) centre (71.8646, -23.3346) ccw
  line L20 (72.3646, -23.3346) -> (72.3646, -28.9894)
  arc A19 (71.8646, -29.4894) -> (72.3646, -28.9894) centre (71.8646, -28.9894) ccw
  line L21 (71.8646, -29.4894) -> (71.5518, -29.4894)
  line L22 (71.5518, -29.4894) -> (71.5518, -38.1)
  line L23 (73.175, -31.1) -> (60.175, -31.1)
  arc A20 (73.675, -31.6) -> (73.175, -31.1) centre (73.175, -31.6) ccw
  line L24 (73.675, -31.6) -> (73.675, -44.6)
  line L25 (60.571, -22.8346) -> (65.667, -22.8346)
  arc A21 (60.571, -22.8346) -> (60.071, -23.3346) centre (60.571, -23.3346) ccw
  line L26 (60.071, -24.138) -> (60.071, -23.3346)
  arc A22 (59.571, -24.638) -> (60.071, -24.138) centre (59.571, -24.138) ccw
  line L27 (59.4026, -24.638) -> (59.571, -24.638)
  arc A23 (59.4026, -24.638) -> (58.9026, -25.138) centre (59.4026, -25.138) ccw
  line L28 (58.9026, -27.186) -> (58.9026, -25.138)
  arc A24 (58.9026, -27.186) -> (59.4026, -27.686) centre (59.4026, -27.186) ccw
  line L29 (59.571, -27.686) -> (59.4026, -27.686)
  arc A25 (60.071, -28.186) -> (59.571, -27.686) centre (59.571, -28.186) ccw
  line L30 (60.071, -29.4894) -> (60.071, -28.186)
  line L31 (60.3584, -29.4894) -> (60.071, -29.4894)
  arc A26 (60.8584, -29.9894) -> (60.3584, -29.4894) centre (60.3584, -29.9894) ccw
  line L32 (60.8584, -38.1) -> (60.8584, -29.9894)
  arc A27 (60.175, -31.1) -> (59.675, -31.6) centre (60.175, -31.6) ccw
  line L33 (59.675, -31.6) -> (59.675, -44.6)
  line L34 (60.8584, -38.1) -> (60.8584, -46.2106)
  arc A28 (59.675, -44.6) -> (60.175, -45.1) centre (60.175, -44.6) ccw
  line L35 (73.175, -45.1) -> (60.175, -45.1)
  line L36 (71.5518, -46.7106) -> (71.5518, -38.1)
  arc A29 (73.175, -45.1) -> (73.675, -44.6) centre (73.175, -44.6) ccw
  arc A30 (60.3584, -46.7106) -> (60.8584, -46.2106) centre (60.3584, -46.2106) ccw
  line L37 (60.3584, -46.7106) -> (60.071, -46.7106)
  line L38 (60.071, -46.7106) -> (60.071, -48.014)
  arc A31 (59.571, -48.514) -> (60.071, -48.014) centre (59.571, -48.014) ccw
  line L39 (59.571, -48.514) -> (59.4026, -48.514)
  arc A32 (59.4026, -48.514) -> (58.9026, -49.014) centre (59.4026, -49.014) ccw
  line L40 (58.9026, -49.014) -> (58.9026, -51.062)
  arc A33 (58.9026, -51.062) -> (59.4026, -51.562) centre (59.4026, -51.062) ccw
  line L41 (59.4026, -51.562) -> (59.571, -51.562)
  arc A34 (60.071, -52.062) -> (59.571, -51.562) centre (59.571, -52.062) ccw
  line L42 (60.071, -52.062) -> (60.071, -52.8654)
  arc A35 (60.071, -52.8654) -> (60.571, -53.3654) centre (60.571, -52.8654) ccw
  line L43 (60.571, -53.3654) -> (65.667, -53.3654)
  arc A36 (66.167, -53.8654) -> (65.667, -53.3654) centre (65.667, -53.8654) ccw
  line L44 (66.167, -53.8654) -> (66.167, -54.229)
  line L45 (66.167, -54.229) -> (68.461, -54.229)
  arc A37 (68.461, -54.229) -> (68.961, -53.729) centre (68.461, -53.729) ccw
  line L46 (68.961, -53.729) -> (68.961, -53.3654)
  line L47 (68.961, -53.3654) -> (71.8646, -53.3654)
  arc A38 (71.8646, -53.3654) -> (72.3646, -52.8654) centre (71.8646, -52.8654) ccw
  line L48 (72.3646, -52.8654) -> (72.3646, -47.2106)
  line L49 (71.8646, -46.7106) -> (71.5518, -46.7106)
  arc A39 (72.3646, -47.2106) -> (71.8646, -46.7106) centre (71.8646, -47.2106) ccw
  line L50 (72.3646, -61.4346) -> (72.3646, -67.0894)
  arc A40 (71.8646, -67.5894) -> (72.3646, -67.0894) centre (71.8646, -67.0894) ccw
  line L51 (71.8646, -67.5894) -> (71.5518, -67.5894)
  line L52 (71.5518, -67.5894) -> (71.5518, -76.2)
  line L53 (73.175, -69.2) -> (60.175, -69.2)
  arc A41 (73.675, -69.7) -> (73.175, -69.2) centre (73.175, -69.7) ccw
  line L54 (73.675, -69.7) -> (73.675, -82.7)
  arc A42 (73.175, -83.2) -> (73.675, -82.7) centre (73.175, -82.7) ccw
  line L55 (71.5518, -84.8106) -> (71.5518, -76.2)
  line L56 (73.175, -83.2) -> (60.175, -83.2)
  line L57 (59.675, -69.7) -> (59.675, -82.7)
  arc A43 (60.175, -69.2) -> (59.675, -69.7) centre (60.175, -69.7) ccw
  arc A44 (59.675, -82.7) -> (60.175, -83.2) centre (60.175, -82.7) ccw
  line L58 (60.8584, -76.2) -> (60.8584, -84.3106)
  line L59 (60.8584, -76.2) -> (60.8584, -68.0894)
  arc A45 (60.8584, -68.0894) -> (60.3584, -67.5894) centre (60.3584, -68.0894) ccw
  line L60 (60.3584, -67.5894) -> (60.071, -67.5894)
  line L61 (60.071, -67.5894) -> (60.071, -66.286)
  arc A46 (60.071, -66.286) -> (59.571, -65.786) centre (59.571, -66.286) ccw
  line L62 (59.571, -65.786) -> (59.4026, -65.786)
  arc A47 (58.9026, -65.286) -> (59.4026, -65.786) centre (59.4026, -65.286) ccw
  line L63 (58.9026, -65.286) -> (58.9026, -63.238)
  arc A48 (59.4026, -62.738) -> (58.9026, -63.238) centre (59.4026, -63.238) ccw
  line L64 (59.4026, -62.738) -> (59.571, -62.738)
  arc A49 (59.571, -62.738) -> (60.071, -62.238) centre (59.571, -62.238) ccw
  line L65 (60.071, -62.238) -> (60.071, -61.4346)
  arc A50 (60.571, -60.9346) -> (60.071, -61.4346) centre (60.571, -61.4346) ccw
  line L66 (60.571, -60.9346) -> (65.667, -60.9346)
  arc A51 (65.667, -60.9346) -> (66.167, -60.4346) centre (65.667, -60.4346) ccw
  line L67 (66.167, -60.4346) -> (66.167, -60.071)
  line L68 (66.167, -60.071) -> (68.461, -60.071)
  arc A52 (68.961, -60.571) -> (68.461, -60.071) centre (68.461, -60.571) ccw
  line L69 (68.961, -60.571) -> (68.961, -60.9346)
  line L70 (68.961, -60.9346) -> (71.8646, -60.9346)
  arc A53 (72.3646, -61.4346) -> (71.8646, -60.9346) centre (71.8646, -61.4346) ccw
  arc A54 (72.3646, -85.3106) -> (71.8646, -84.8106) centre (71.8646, -85.3106) ccw
  line L71 (71.8646, -84.8106) -> (71.5518, -84.8106)
  line L72 (72.3646, -90.9654) -> (72.3646, -85.3106)
  arc A55 (71.8646, -91.4654) -> (72.3646, -90.9654) centre (71.8646, -90.9654) ccw
  line L73 (68.961, -91.4654) -> (71.8646, -91.4654)
  line L74 (68.961, -91.829) -> (68.961, -91.4654)
  arc A56 (68.461, -92.329) -> (68.961, -91.829) centre (68.461, -91.829) ccw
  line L75 (66.167, -92.329) -> (68.461, -92.329)
  line L76 (66.167, -91.9654) -> (66.167, -92.329)
  arc A57 (66.167, -91.9654) -> (65.667, -91.4654) centre (65.667, -91.9654) ccw
  line L77 (60.571, -91.4654) -> (65.667, -91.4654)
  arc A58 (60.071, -90.9654) -> (60.571, -91.4654) centre (60.571, -90.9654) ccw
  line L78 (60.071, -90.162) -> (60.071, -90.9654)
  arc A59 (60.071, -90.162) -> (59.571, -89.662) centre (59.571, -90.162) ccw
  arc A60 (58.9026, -89.162) -> (59.4026, -89.662) centre (59.4026, -89.162) ccw
  line L79 (59.4026, -89.662) -> (59.571, -89.662)
  line L80 (58.9026, -87.114) -> (58.9026, -89.162)
  arc A61 (59.4026, -86.614) -> (58.9026, -87.114) centre (59.4026, -87.114) ccw
  line L81 (59.571, -86.614) -> (59.4026, -86.614)
  arc A62 (59.571, -86.614) -> (60.071, -86.114) centre (59.571, -86.114) ccw
  line L82 (60.071, -84.8106) -> (60.071, -86.114)
  line L83 (60.3584, -84.8106) -> (60.071, -84.8106)
  arc A63 (60.3584, -84.8106) -> (60.8584, -84.3106) centre (60.3584, -84.3106) ccw
  line L84 (2.525, -22.075) -> (2.525, -35.075)
  line L85 (3.025, -21.575) -> (16.025, -21.575)
  arc A64 (3.025, -21.575) -> (2.525, -22.075) centre (3.025, -22.075) ccw
  arc A65 (16.525, -22.075) -> (16.025, -21.575) centre (16.025, -22.075) ccw
  line L86 (16.525, -22.075) -> (16.525, -35.075)
  arc A66 (16.025, -35.575) -> (16.525, -35.075) centre (16.025, -35.075) ccw
  line L87 (3.025, -35.575) -> (16.025, -35.575)
  arc A67 (2.525, -35.075) -> (3.025, -35.575) centre (3.025, -35.075) ccw
  line L88 (22.075, -35.575) -> (35.075, -35.575)
  arc A68 (21.575, -35.075) -> (22.075, -35.575) centre (22.075, -35.075) ccw
  line L89 (21.575, -22.075) -> (21.575, -35.075)
  arc A69 (22.075, -21.575) -> (21.575, -22.075) centre (22.075, -22.075) ccw
  line L90 (22.075, -21.575) -> (35.075, -21.575)
  arc A70 (35.575, -22.075) -> (35.075, -21.575) centre (35.075, -22.075) ccw
  line L91 (35.575, -22.075) -> (35.575, -35.075)
  arc A71 (35.075, -35.575) -> (35.575, -35.075) centre (35.075, -35.075) ccw
  line L92 (40.625, -22.075) -> (40.625, -35.075)
  arc A72 (40.625, -35.075) -> (41.125, -35.575) centre (41.125, -35.075) ccw
  line L93 (41.125, -35.575) -> (54.125, -35.575)
  arc A73 (41.125, -21.575) -> (40.625, -22.075) centre (41.125, -22.075) ccw
  line L94 (41.125, -21.575) -> (54.125, -21.575)
  arc A74 (54.625, -22.075) -> (54.125, -21.575) centre (54.125, -22.075) ccw
  line L95 (54.625, -22.075) -> (54.625, -35.075)
  arc A75 (54.125, -35.575) -> (54.625, -35.075) centre (54.125, -35.075) ccw
  line L96 (41.125, -40.625) -> (54.125, -40.625)
  line L97 (41.125, -54.625) -> (54.125, -54.625)
  arc A76 (54.125, -54.625) -> (54.625, -54.125) centre (54.125, -54.125) ccw
  line L98 (54.625, -41.125) -> (54.625, -54.125)
  arc A77 (54.625, -41.125) -> (54.125, -40.625) centre (54.125, -41.125) ccw
  arc A78 (41.125, -40.625) -> (40.625, -41.125) centre (41.125, -41.125) ccw
  line L99 (40.625, -41.125) -> (40.625, -54.125)
  arc A79 (40.625, -54.125) -> (41.125, -54.625) centre (41.125, -54.125) ccw
  line L100 (22.075, -40.625) -> (35.075, -40.625)
  line L101 (35.575, -41.125) -> (35.575, -54.125)
  line L102 (22.075, -54.625) -> (35.075, -54.625)
  line L103 (21.575, -41.125) -> (21.575, -54.125)
  arc A80 (21.575, -54.125) -> (22.075, -54.625) centre (22.075, -54.125) ccw
  arc A81 (35.075, -54.625) -> (35.575, -54.125) centre (35.075, -54.125) ccw
  arc A82 (35.575, -41.125) -> (35.075, -40.625) centre (35.075, -41.125) ccw
  arc A83 (22.075, -40.625) -> (21.575, -41.125) centre (22.075, -41.125) ccw
  line L104 (3.025, -40.625) -> (16.025, -40.625)
  line L105 (16.525, -41.125) -> (16.525, -54.125)
  line L106 (2.525, -41.125) -> (2.525, -54.125)
  line L107 (3.025, -54.625) -> (16.025, -54.625)
  arc A84 (2.525, -54.125) -> (3.025, -54.625) centre (3.025, -54.125) ccw
  arc A85 (16.025, -54.625) -> (16.525, -54.125) centre (16.025, -54.125) ccw
  arc A86 (16.525, -41.125) -> (16.025, -40.625) centre (16.025, -41.125) ccw
  arc A87 (3.025, -40.625) -> (2.525, -41.125) centre (3.025, -41.125) ccw
  line L108 (3.025, -59.675) -> (16.025, -59.675)
  line L109 (16.525, -60.175) -> (16.525, -73.175)
  line L110 (2.525, -60.175) -> (2.525, -73.175)
  line L111 (3.025, -73.675) -> (16.025, -73.675)
  arc A88 (2.525, -73.175) -> (3.025, -73.675) centre (3.025, -73.175) ccw
  arc A89 (16.025, -73.675) -> (16.525, -73.175) centre (16.025, -73.175) ccw
  arc A90 (16.525, -60.175) -> (16.025, -59.675) centre (16.025, -60.175) ccw
  arc A91 (3.025, -59.675) -> (2.525, -60.175) centre (3.025, -60.175) ccw
  line L112 (22.075, -59.675) -> (35.075, -59.675)
  line L113 (21.575, -60.175) -> (21.575, -73.175)
  arc A92 (22.075, -59.675) -> (21.575, -60.175) centre (22.075, -60.175) ccw
  arc A93 (35.575, -60.175) -> (35.075, -59.675) centre (35.075, -60.175) ccw
  line L114 (35.575, -60.175) -> (35.575, -73.175)
  line L115 (22.075, -73.675) -> (35.075, -73.675)
  arc A94 (35.075, -73.675) -> (35.575, -73.175) centre (35.075, -73.175) ccw
  arc A95 (21.575, -73.175) -> (22.075, -73.675) centre (22.075, -73.175) ccw
  line L116 (41.125, -73.675) -> (54.125, -73.675)
  arc A96 (40.625, -73.175) -> (41.125, -73.675) centre (41.125, -73.175) ccw
  line L117 (40.625, -60.175) -> (40.625, -73.175)
  line L118 (54.625, -60.175) -> (54.625, -73.175)
  arc A97 (54.125, -73.675) -> (54.625, -73.175) centre (54.125, -73.175) ccw
  arc A98 (54.625, -60.175) -> (54.125, -59.675) centre (54.125, -60.175) ccw
  line L119 (41.125, -59.675) -> (54.125, -59.675)
  arc A99 (41.125, -59.675) -> (40.625, -60.175) centre (41.125, -60.175) ccw
  line L120 (41.125, -78.725) -> (54.125, -78.725)
  arc A100 (54.625, -79.225) -> (54.125, -78.725) centre (54.125, -79.225) ccw
  line L121 (54.625, -79.225) -> (54.625, -92.225)
  arc A101 (54.125, -92.725) -> (54.625, -92.225) centre (54.125, -92.225) ccw
  line L122 (41.125, -92.725) -> (54.125, -92.725)
  arc A102 (40.625, -92.225) -> (41.125, -92.725) centre (41.125, -92.225) ccw
  line L123 (40.625, -79.225) -> (40.625, -92.225)
  arc A103 (41.125, -78.725) -> (40.625, -79.225) centre (41.125, -79.225) ccw
  line L124 (33.8154, -80.0354) -> (28.1606, -80.0354)
  arc A104 (34.3154, -80.5354) -> (33.8154, -80.0354) centre (33.8154, -80.5354) ccw
  line L125 (34.3154, -83.439) -> (34.3154, -80.5354)
  arc A105 (28.1606, -80.0354) -> (27.6606, -80.5354) centre (28.1606, -80.5354) ccw
  line L126 (27.6606, -80.8482) -> (19.05, -80.8482)
  line L127 (27.6606, -80.5354) -> (27.6606, -80.8482)
  line L128 (34.679, -83.439) -> (34.3154, -83.439)
  arc A106 (35.179, -83.939) -> (34.679, -83.439) centre (34.679, -83.939) ccw
  line L129 (35.179, -86.233) -> (35.179, -83.939)
  line L130 (34.8154, -86.233) -> (35.179, -86.233)
  arc A107 (34.8154, -86.233) -> (34.3154, -86.733) centre (34.8154, -86.733) ccw
  line L131 (34.3154, -91.829) -> (34.3154, -86.733)
  arc A108 (33.8154, -92.329) -> (34.3154, -91.829) centre (33.8154, -91.829) ccw
  line L132 (33.012, -92.329) -> (33.8154, -92.329)
  arc A109 (33.012, -92.329) -> (32.512, -92.829) centre (33.012, -92.829) ccw
  line L133 (32.512, -92.9974) -> (32.512, -92.829)
  arc A110 (32.012, -93.4974) -> (32.512, -92.9974) centre (32.012, -92.9974) ccw
  line L134 (29.964, -93.4974) -> (32.012, -93.4974)
  arc A111 (29.464, -92.9974) -> (29.964, -93.4974) centre (29.964, -92.9974) ccw
  line L135 (29.464, -92.829) -> (29.464, -92.9974)
  arc A112 (29.464, -92.829) -> (28.964, -92.329) centre (28.964, -92.829) ccw
  line L136 (27.6606, -92.329) -> (28.964, -92.329)
  line L137 (27.6606, -92.0416) -> (27.6606, -92.329)
  arc A113 (27.6606, -92.0416) -> (27.1606, -91.5416) centre (27.1606, -92.0416) ccw
  line L138 (19.05, -91.5416) -> (27.1606, -91.5416)
  line L139 (26.05, -79.225) -> (26.05, -92.225)
  arc A114 (25.55, -92.725) -> (26.05, -92.225) centre (25.55, -92.225) ccw
  line L140 (12.55, -92.725) -> (25.55, -92.725)
  line L141 (19.05, -91.5416) -> (10.9394, -91.5416)
  arc A115 (12.05, -92.225) -> (12.55, -92.725) centre (12.55, -92.225) ccw
  line L142 (12.05, -79.225) -> (12.05, -92.225)
  line L143 (12.55, -78.725) -> (25.55, -78.725)
  arc A116 (26.05, -79.225) -> (25.55, -78.725) centre (25.55, -79.225) ccw
  arc A117 (12.55, -78.725) -> (12.05, -79.225) centre (12.55, -79.225) ccw
  line L144 (10.4394, -80.8482) -> (19.05, -80.8482)
  arc A118 (10.4394, -80.5354) -> (9.9394, -80.0354) centre (9.9394, -80.5354) ccw
  line L145 (10.4394, -80.5354) -> (10.4394, -80.8482)
  line L146 (4.2846, -80.0354) -> (9.9394, -80.0354)
  arc A119 (4.2846, -80.0354) -> (3.7846, -80.5354) centre (4.2846, -80.5354) ccw
  line L147 (3.7846, -83.439) -> (3.7846, -80.5354)
  arc A120 (3.421, -83.439) -> (2.921, -83.939) centre (3.421, -83.939) ccw
  line L148 (3.421, -83.439) -> (3.7846, -83.439)
  line L149 (2.921, -86.233) -> (2.921, -83.939)
  line L150 (3.2846, -86.233) -> (2.921, -86.233)
  arc A121 (3.7846, -86.733) -> (3.2846, -86.233) centre (3.2846, -86.733) ccw
  line L151 (3.7846, -91.829) -> (3.7846, -86.733)
  arc A122 (3.7846, -91.829) -> (4.2846, -92.329) centre (4.2846, -91.829) ccw
  line L152 (5.088, -92.329) -> (4.2846, -92.329)
  arc A123 (5.588, -92.829) -> (5.088, -92.329) centre (5.088, -92.829) ccw
  line L153 (5.588, -92.9974) -> (5.588, -92.829)
  arc A124 (5.588, -92.9974) -> (6.088, -93.4974) centre (6.088, -92.9974) ccw
  line L154 (8.136, -93.4974) -> (6.088, -93.4974)
  arc A125 (8.136, -93.4974) -> (8.636, -92.9974) centre (8.136, -92.9974) ccw
  arc A126 (9.136, -92.329) -> (8.636, -92.829) centre (9.136, -92.829) ccw
  line L155 (8.636, -92.829) -> (8.636, -92.9974)
  line L156 (10.4394, -92.329) -> (9.136, -92.329)
  line L157 (10.4394, -92.0416) -> (10.4394, -92.329)
  arc A127 (10.9394, -91.5416) -> (10.4394, -92.0416) centre (10.9394, -92.0416) ccw
  line L158 (-5, -87.25) -> (-5, -79.25)
  arc A128 (-3, -77.25) -> (-5, -79.25) centre (-3, -79.25) ccw
  line L159 (-3, -77.25) -> (0, -77.25)
  arc A129 (-5, -87.25) -> (-3, -89.25) centre (-3, -87.25) ccw
  line L160 (0, -89.25) -> (-3, -89.25)
  line L161 (0, -95.25) -> (76.2, -95.25)
  circle A130 centre (-2.5, -83.25) radius 1.7
  line L162 (-3, -25.25) -> (0, -25.25)
  arc A131 (-3, -25.25) -> (-5, -27.25) centre (-3, -27.25) ccw
  line L163 (-5, -35.25) -> (-5, -27.25)
  arc A132 (-5, -35.25) -> (-3, -37.25) centre (-3, -35.25) ccw
  line L164 (0, -37.25) -> (-3, -37.25)
  circle A133 centre (-2.5, -31.25) radius 1.7
  line L165 (0, 3.431) -> (-3, 3.431)
  arc A134 (-5, 5.431) -> (-3, 3.431) centre (-3, 5.431) ccw
  line L166 (-5, 5.431) -> (-5, 13.431)
  circle A135 centre (-2.5, 9.431) radius 1.7
  line L167 (-3, 15.431) -> (0, 15.431)
  arc A136 (-3, 15.431) -> (-5, 13.431) centre (-3, 13.431) ccw
  line L168 (76.2, 21.431) -> (0, 21.431)
  line L169 (76.2, 15.431) -> (79.2, 15.431)
  arc A137 (81.2, 13.431) -> (79.2, 15.431) centre (79.2, 13.431) ccw
  line L170 (81.2, 13.431) -> (81.2, 5.431)
  arc A138 (79.2, 3.431) -> (81.2, 5.431) centre (79.2, 5.431) ccw
  line L171 (79.2, 3.431) -> (76.2, 3.431)
  circle A139 centre (78.7, 9.431) radius 1.7
  line L172 (76.2, -25.25) -> (79.2, -25.25)
  arc A140 (81.2, -27.25) -> (79.2, -25.25) centre (79.2, -27.25) ccw
  line L173 (81.2, -27.25) -> (81.2, -35.25)
  circle A141 centre (78.7, -31.25) radius 1.7
  arc A142 (79.2, -37.25) -> (81.2, -35.25) centre (79.2, -35.25) ccw
  line L174 (79.2, -37.25) -> (76.2, -37.25)
  line L175 (81.2, -79.25) -> (81.2, -87.25)
  arc A143 (81.2, -79.25) -> (79.2, -77.25) centre (79.2, -79.25) ccw
  line L176 (79.2, -77.25) -> (76.2, -77.25)
  line L177 (76.2, -89.25) -> (79.2, -89.25)
  arc A144 (79.2, -89.25) -> (81.2, -87.25) centre (79.2, -87.25) ccw
  circle A145 centre (78.7, -83.25) radius 1.7
  line L178 (77.7, -25.25) -> (77.7, 3.431)
  line L179 (77.7, 15.431) -> (77.7, 24.3133)
  line L180 (-1.5, 15.431) -> (-1.5, 28.3642)
  line L181 (-1.5, 3.431) -> (-1.5, -25.25)
  line L182 (-1.5, -37.25) -> (-1.5, -77.25)
  line L183 (-1.5, -89.25) -> (-1.5, -98.79)
  line L184 (77.7, -89.25) -> (77.7, -99.5266)
  line L185 (77.7, -77.25) -> (77.7, -37.25)
  line L186 (0, -95.25) -> (-1.5, -95.25)
  line L187 (76.2, -95.25) -> (77.7, -95.25)
  line L188 (76.2, 21.431) -> (77.7, 21.431)
  line L189 (0, 21.431) -> (-1.5, 21.431)
  point P0 (16.025, -3.025)
  point P1 (16.025, -35.575)
  constraint midpoint L172 L178.start
  constraint midpoint L171 L178.end
  constraint midpoint L169 L179.start
  constraint perpendicular L169 L179
  constraint midpoint L167 L180.start
  constraint perpendicular L167 L180
  constraint midpoint L165 L181.start
  constraint midpoint L162 L181.end
  constraint midpoint L164 L182.start
  constraint midpoint L159 L182.end
  constraint midpoint L160 L183.start
  constraint perpendicular L160 L183
  constraint midpoint L177 L184.start
  constraint perpendicular L177 L184
  constraint midpoint L176 L185.start
  constraint midpoint L174 L185.end
  constraint coincident L161.start L186.start
  constraint coincident L183 L186.end
  constraint perpendicular L183 L186
  constraint coincident L161.end L187.start
  constraint coincident L184 L187.end
  constraint perpendicular L184 L187
  constraint coincident L168.start L188.start
  constraint coincident L179 L188.end
  constraint perpendicular L179 L188
  constraint coincident L168.end L189.start
  constraint coincident L180 L189.end
  constraint perpendicular L180 L189
extrude "Extrude1" add sketch "Sketch4" along normal blind 1.5
equation "d3 = d2"
equation "d4 = d5"
equation "d9 = d2 / 2"
equation "d11 = d6"
equation "d12 = d8"
equation "d13 = d3 / 2"
equation "d14 = d11 / 2"
equation "d15 = d6 / 2"
equation "d16 = d6"
equation "d17 = d6"
equation "d18 = d7"
equation "d19 = d7"
equation "d20 = d8"
equation "d21 = d3 / 2"
equation "d22 = d16 / 2"
equation "d23 = d20"
equation "d24 = d17 / 2"
equation "d25 = d9"
equation "d26 = d11"
equation "d27 = d12"
equation "d28 = d26"
equation "d29 = d27"
equation "d30 = d3 / 2"
equation "d31 = d26 / 2"
equation "d32 = d2 / 2"
equation "d33 = d28 / 2"
